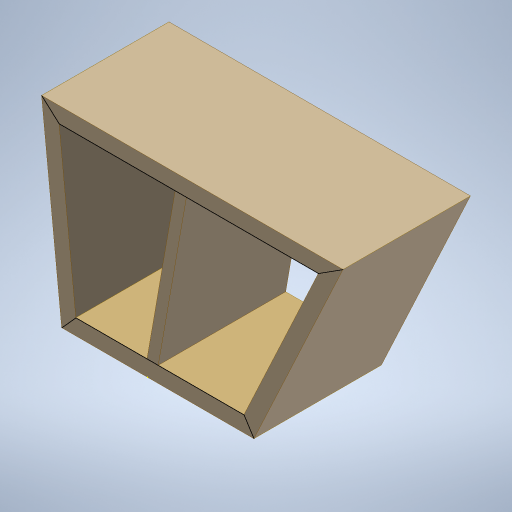
# Autodesk Inventor part: Slant Box
Saved by Autodesk Inventor 2024 (Build 280153000, 153)
## iProperties
Created: 2014-05-28
Part Number: Slant Box
Material: Generic
Document SubType Name: Modeling
Designer: SauliusD
Density: 1 g/cm^3
Appearance: Default
Description: Slant Box
Author: SauliusD
Autodesk Inventor part; units mm, degrees
ref_plane "YZ Plane" through (0, 0, 0) normal (1, 0, 0) x (0, 1, 0)
ref_plane "XZ Plane" through (0, 0, 0) normal (0, 1, 0) x (-1, 0, 0)
ref_plane "XY Plane" through (0, 0, 0) normal (0, 0, 1) x (1, 0, 0)
sketch "Sketch1" plane through (0, 0, 0) normal (0, 0, 1) x (1, 0, 0)
  line L0 (-250, -150) -> (250, -150)
  line L1 (250, -150) -> (250, 150)
  line L2 (250, 150) -> (-250, 150)
  line L3 (-250, 150) -> (-250, -150)
  line L4 (-250, -150) -> (250, 150) construction
  line L5 (250, -150) -> (-250, 150) construction
  point P0 (0, 0)
  dimension "d0" = 500
  dimension "d1" = 300
  constraints: 12 end point, 2 midpoint, 2 parallel, 1 horizontal, 1 perpendicular
  measures "d0" distance of L2.end L1.end
  measures "d1" distance of L1.end L0.end
extrude "Extrusion1" add sketch "Sketch1" along normal blind 450
draft "FaceDraft1" angle 25 pull direction (0, 0, -1) faces at (250, -50, 150) fixed edges at (250, 0, 0)
draft "FaceDraft2" angle 6 pull direction (0, 0, -1) faces at (-250, 50, 150) fixed edges at (-250, 0, 450)
shell "Shell1" thickness 37 removed faces 2 at (153.2795, -150, 300) at (153.2795, 150, 300)
sketch "Sketch2" plane through (-202.7031, -150, 0) normal (0, -1, 0) x (1, 0, 0)
  line L0 (-6.2042, 413) -> (604.4632, 413) construction
  line L1 (-47.2969, 450) -> (-6.2042, 413)
  line L2 (-6.2042, 413) -> (604.4632, 413)
  line L3 (604.4632, 413) -> (662.5415, 450)
  line L4 (0, 0) -> (33.3149, 37)
  line L5 (33.3149, 37) -> (429.1315, 37)
  line L6 (429.1315, 37) -> (452.7031, 0)
  point P0 (202.7031, 0)
  constraints: 12 end point, 1 collinear, 1 parallel, 1 perpendicular
surface extrude "ExtrusionSrf1" sketch "Sketch2" against normal up to surface (300 mm away) shown yes curves L1 L2 L3
surface extrude "ExtrusionSrf2" sketch "Sketch2" against normal up to surface (300 mm away) shown yes curves L4 L5 L6
split body "Split1" sketch "Sketch2" result two bodies curves L1 L2 L3 first body at (-13.3872, 50, 449.5)
split body "Split2" result two bodies by surface "ExtrusionSrf2" bodies 3 first body at (99.099, -50, 0.5)
sketch "Sketch3" plane through (-250, -150, 450) normal (0, -1, 0) x (1, 0, 0)
  line L0 (314.6185, -37) -> (341.0196, -37)
  line L1 (341.0196, -37) -> (274.7206, -413)
  line L2 (80.6119, -413) -> (476.4284, -413) projected
  line L3 (248.3195, -413) -> (314.6185, -37)
  line L4 (41.0927, -37) -> (651.7601, -37) projected
  line L5 (651.7601, -37) -> (476.4284, -413) projected
  point P0 (250, -450)
  dimension "d11" = 26
  dimension "d14" = 80
  constraints: 6 end point, 2 point on line, 1 collinear, 1 horizontal, 1 parallel
  measures "d11" distance between parallel lines of L1 L3
  measures "d14" angle of L2 L1
extrude "Extrusion2" add sketch "Sketch3" against normal up to surface (300 mm away) separate body contours L0 L1 L2 L3
body "Srf1"
body "Srf2"
